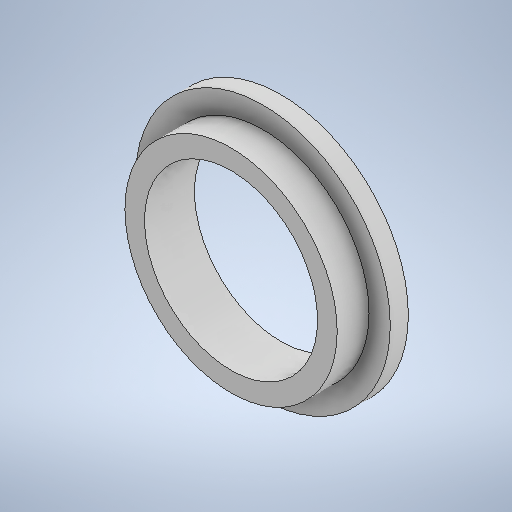
# Autodesk Inventor part: Bushing
Saved by Autodesk Inventor 2025.1 (Build 291241000, 241)
## iProperties
Created: 2025-05-20
Part Number: Bushing
Material: Generic
Document SubType Name: Modeling
Designer: Andreas' PC
Density: 1 g/cm^3
Appearance: Default
Author: Andreas' PC
Autodesk Inventor part; units mm, degrees
ref_plane "YZ Plane" through (0, 0, 0) normal (1, 0, 0) x (0, 1, 0)
ref_plane "XZ Plane" through (0, 0, 0) normal (0, 1, 0) x (-1, 0, 0)
ref_plane "XY Plane" through (0, 0, 0) normal (0, 0, 1) x (1, 0, 0)
sketch "Sketch1" plane through (0, 0, 0) normal (0, 0, 1) x (1, 0, 0)
  circle A0 centre (0, 0) radius 8.15
  circle A1 centre (0, 0) radius 10
  circle A2 centre (0, 0) radius 12
  dimension "d0" = 16.3
  dimension "d1" = 20
  dimension "d2" = 24
  constraints: 3 centre point, 3 coincident
  measures "d0" diameter of A0
  measures "d1" diameter of A1
  measures "d2" diameter of A2
extrude "Extrusion1" add sketch "Sketch1" along normal blind 4.7 contours A1
extrude "Extrusion2" add sketch "Sketch1" along normal blind 1.7 contours A2
equation "\"d0\" = inner_d"
equation "\"d1\" = outer_d"
equation "\"d5\" = spacing"
equation "\"inner_d\" = 16.3"
equation "\"outer_d\" = 20"
equation "\"spacing\" = 1.7"
body "Solid1"
